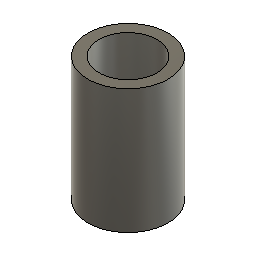
feet (Autodesk Fusion 360 design; units mm, degrees)
Autodesk Fusion 360 part; units mm, degrees
sketch "Sketch1" plane through (0, 0, 0) normal (0, 1, 0) x (1, 0, 0)
  circle A0 centre (0, 0) radius 1.75
  circle A1 centre (0, 0) radius 3.25
  circle A2 centre (0, 0) radius 4.5
  dimension "d1" = 3.5
  dimension "d2" = 6.5
  dimension "d3" = 9
  constraint coincident A0.centre A1.centre
  constraint concentric A0 A2
  measures "d1" diameter of A0
  measures "d2" diameter of A1
  measures "d3" diameter of A2
extrude "Extrude1" add sketch "Sketch1" along normal blind 14 contours A2
sketch "Sketch2" plane through (0, 0, 0) normal (0, 1, 0) x (1, 0, 0)
  circle A0 centre (0, 0) radius 1.75
  circle A1 centre (0, 0) radius 3.25
  dimension "d6" = 3.5
  dimension "d7" = 6.5
  constraint coincident A0.centre A1.centre
  constraint concentric A0 A1
  measures "d6" diameter of A0
  measures "d7" diameter of A1
extrude "Extrude2" add sketch "Sketch2" along normal blind 2
